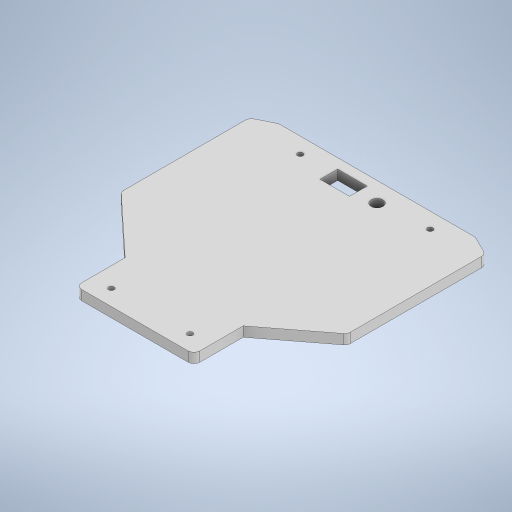
# Autodesk Inventor part: DeTren
Saved by Autodesk Inventor 2023 (Build 270158000, 158)
## iProperties
Created: 2023-03-06
Part Number: DeTren
Material: Generic
Document SubType Name: Modeling
Designer: Admins
Density: 1 g/cm^3
Appearance: Default
Author: Admins
Autodesk Inventor part; units mm, degrees
ref_plane "YZ Plane" through (0, 0, 0) normal (1, 0, 0) x (0, 1, 0)
ref_plane "XZ Plane" through (0, 0, 0) normal (0, 1, 0) x (-1, 0, 0)
ref_plane "XY Plane" through (0, 0, 0) normal (0, 0, 1) x (1, 0, 0)
sketch "Sketch1" plane through (0, 0, 0) normal (0, 1, 0) x (-1, 0, 0)
  line L0 (60, -75) -> (-60, -75)
  line L1 (-60, 75) -> (60, -75) construction
  line L2 (60, 75) -> (-60, -75) construction
  line L3 (-60, -75) -> (-60, -55)
  line L4 (-60, -42.5) -> (-60, -55)
  line L5 (0, 75) -> (0, 40)
  line L6 (-60, -75) -> (-60, -5)
  line L7 (-30, 40) -> (-30, 10)
  line L8 (-30, 10) -> (-60, 0)
  line L9 (30, 40) -> (30, 10)
  line L10 (30, 10) -> (60, -5)
  line L11 (-30, 40) -> (-30, 48)
  line L12 (30, 40) -> (30, 48)
  line L13 (0, 75) -> (0, -75)
  line L14 (0, -75) -> (-60, -75)
  line L15 (60, -70) -> (60, -55)
  line L16 (60, -42.5) -> (60, -55)
  line L17 (60, -5) -> (60, -70)
  line L18 (-60, -75) -> (-60, 0)
  line L19 (57, -75) -> (50, -75)
  line L20 (60, -70) -> (60, -75)
  line L21 (-60, -75) -> (-50, -75)
  line L22 (-60, -70) -> (-60, -75)
  line L23 (-60, -70) -> (-50, -75)
  line L24 (60, -70) -> (50, -75)
  line L25 (-27.5, -75) -> (27.5, -75)
  line L26 (27.5, -75) -> (27.5, -5)
  line L27 (27.5, -5) -> (-27.5, -5)
  line L28 (-27.5, -5) -> (-27.5, -75)
  line L29 (30, 10) -> (-30, 10)
  line L30 (0, 75) -> (0, 40)
  line L31 (0, 40) -> (20, 40)
  line L32 (20, 40) -> (-20, 40)
  circle A0 centre (20, 40) radius 1.4
  circle A1 centre (-20, 40) radius 1.4
  line L33 (30, 48) -> (-30, 48)
  line L34 (-60, -75) -> (-35, -75)
  line L35 (60, -75) -> (35, -75)
  line L36 (35, -75) -> (31, -75)
  line L37 (31, -75) -> (31, -67)
  line L38 (31, -67) -> (35, -67)
  line L39 (35, -67) -> (35, -75)
  line L40 (-35, -75) -> (-39, -75)
  line L41 (-39, -75) -> (-39, -67)
  line L42 (-39, -67) -> (-35, -67)
  line L43 (-35, -67) -> (-35, -75)
  circle A2 centre (-35, -67) radius 1.4
  circle A3 centre (31, -67) radius 1.4
  line L44 (30, 48) -> (30, 23)
  line L45 (30, 23) -> (60, -5)
  line L46 (-30, 48) -> (-30, 23)
  line L47 (-30, 23) -> (-60, 0)
  dimension "d0" = 120
  dimension "d1" = 150
  dimension "d18" = 70
  dimension "d43" = 55
  dimension "d44" = 70
  dimension "d45" = 35
  dimension "d46" = 20
  dimension "d47" = 40
  dimension "d48" = 2.8
  dimension "d49" = 2.8
  dimension "d50" = 25
  dimension "d51" = 25
  dimension "d52" = 4
  dimension "d53" = 8
  dimension "d54" = 4
  dimension "d55" = 8
  dimension "d56" = 2.8
  dimension "d57" = 2.8
  dimension "d73" = 25
  dimension "d74" = 25
  constraints: 96 end point, 10 point on line, 9 parallel, 5 horizontal, 4 centre point, 4 coincident, 4 perpendicular, 2 vertical, 1 collinear, 1 midpoint
  measures "d0" distance of L1.end L2.end
  measures "d1" distance of L2.start L1.end
  measures "d18" distance of L2.end L6.end
  measures "d43" distance of L27.end L26.end
  measures "d44" distance of L26.end L25.end
  measures "d45" distance of L13.start L5.end
  measures "d46" distance of L5.end L31.end
  measures "d47" distance of L31.end L32.end
  measures "d48" diameter of A0
  measures "d49" diameter of A1
  measures "d50" distance of L2.end L34.end
  measures "d51" distance of L1.end L35.end
  measures "d52" distance of L37.end L38.end
  measures "d53" distance of L36.end L37.end
  measures "d54" distance of L41.end L42.end
  measures "d55" distance of L40.end L41.end
  measures "d56" diameter of A2
  measures "d57" diameter of A3
  measures "d73" distance of L12.end L44.end
  measures "d74" distance of L11.end L46.end
extrude "Extrusion1" add sketch "Sketch1" along normal blind 5 contours L24 L0 L39 L38 A3 L37 L26 L27 L13 L29 L10 L17 L16 L15 | L0 L37 A3 L38 L39 | L10 L9 L45 | L0 L13 L27 L26 | L29 L13 L5 L33 L12 L9 | L0 L28 L27 L13 | L29 L7 L11 L33 L5 L13 | L13 L27 L28 L0 L43 A2 L42 L41 L23 L3 L4 L6 L18 L8 L29 | L8 L47 L7 | L0 L41 L42 A2 L43
fillet "Fillet1" radius 3 8 edges at (30, 2.5, 48) (60, 2.5, 0) (50, 2.5, -75) (60, 2.5, -70) (-60, 2.5, -70) (-50, 2.5, -75) (-60, 2.5, -5) (-30, 2.5, 48)
sketch "Sketch2" plane through (0, 5, 0) normal (0, 1, 0) x (1, 0, 0)
  line L0 (49.2918, 75) -> (-49.2918, 75) construction
  line L1 (0, 75) -> (0, 65) construction
  line L2 (0, 65) -> (10, 65) construction
  circle A0 centre (10, 65) radius 3
  line L3 (0, 75) -> (0, 70)
  line L4 (0, 75) -> (5, 75) construction
  line L5 (0, 58) -> (0, 70)
  line L6 (0, 70) -> (-15, 70)
  line L7 (-15, 70) -> (-15, 61)
  line L8 (-15, 61) -> (0, 61)
  line L9 (0, 61) -> (0, 70)
  line L10 (0, 75) -> (0, 55)
  point P0 (0, 0)
  dimension "d61" = 10
  dimension "d62" = 10
  dimension "d63" = 6
  dimension "d64" = 5
  dimension "d65" = 90
  dimension "d68" = 15
  dimension "d69" = 9
  dimension "d72" = 20
  constraints: 20 end point, 3 horizontal, 2 parallel, 2 perpendicular, 1 centre point, 1 coincident, 1 collinear, 1 midpoint, 1 point on line, 1 vertical
  measures "d61" distance of L1.start L1.end
  measures "d62" distance of L1.end L2.end
  measures "d63" diameter of A0
  measures "d64" distance of L1.start L3.end
  measures "d65" angle of L3 L4
  measures "d68" distance of L8.end L7.end
  measures "d69" distance of L7.end L6.end
  measures "d72" distance of L1.start L10.end
extrude "Extrusion2" cut sketch "Sketch2" against normal through all
body "Solid1"
